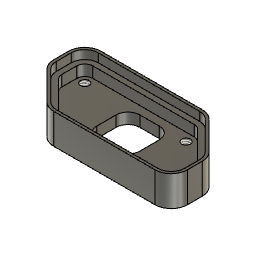
Program and Verify - Challenge (Autodesk Fusion 360 design; units mm, degrees)
Autodesk Fusion 360 part; units mm, degrees
sketch "Sketch1" plane through (0, 0, 0) normal (0, 0, 1) x (1, 0, 0)
  line L0 (47.625, -22.225) -> (-47.625, -22.225)
  line L1 (-47.625, -22.225) -> (-47.625, 22.225)
  line L2 (-47.625, 22.225) -> (47.625, 22.225)
  line L3 (47.625, 22.225) -> (47.625, -22.225)
  line L4 (47.625, -22.225) -> (-47.625, 22.225) construction
  line L5 (-47.625, -22.225) -> (47.625, 22.225) construction
  dimension "d7_1" = 95.25
  dimension "d8_1" = 44.45
  constraint horizontal L0
  constraint perpendicular L0 L1
  constraint parallel L0 L2
  constraint parallel L1 L3
  constraint coincident L4 origin
  constraint coincident L5 origin
  measures "d7_1" distance of L1.end L2.end
  measures "d8_1" distance of L0.end L1.end
extrude "Extrude1" add sketch "Sketch1" along normal blind 17.78
sketch "Sketch2" plane through (0, 0, 17.78) normal (0, 0, 1) x (-1, 0, 0)
  line L0 (-47.625, -22.225) -> (47.625, -22.225)
  line L1 (47.625, -22.225) -> (47.625, 22.225)
  line L2 (47.625, 22.225) -> (-47.625, 22.225)
  line L3 (-47.625, 22.225) -> (-47.625, -22.225)
  line L4 (47.625, 0) -> (25.4, -22.225) construction
  line L5 (-47.625, 0) -> (-25.4, 22.225) construction
  line L6 (47.625, 0) -> (25.4, 22.225)
  line L7 (-47.625, 0) -> (-25.4, -22.225)
  dimension "d11_1" = 45
  dimension "d12_1" = 45
  dimension "d19_1" = 45
  dimension "d20_1" = 45
  constraint midpoint L1 L4.start
  constraint coincident L0 L4.end
  constraint midpoint L3 L5.start
  constraint coincident L2 L5.end
  constraint coincident L2 L6.end
  constraint coincident L0 L7.end
  measures "d11_1" angle of L1 L4
  measures "d12_1" angle of L3 L5
  measures "d19_1" angle of L3 L7
  measures "d20_1" angle of L1 L6
extrude "Extrude2" cut sketch "Sketch2" against normal through all contours L0 L3 L7 | L1 L2 L6
fillet "Fillet1" radius 9.525 6 edges at (-47.625, 0, 8.89) (-25.4, -22.225, 8.89) (47.625, -22.225, 8.89) (47.625, 0, 8.89) (25.4, 22.225, 8.89) (-47.625, 22.225, 8.89)
sketch "Sketch3" plane through (0, 0, 17.78) normal (0, 0, 1) x (-1, 0, 0)
  arc A0 (38.1, -22.225) -> (47.625, -12.7) centre (38.1, -12.7) ccw
  line L0 (47.625, -12.7) -> (47.625, -3.9454)
  arc A1 (47.625, -3.9454) -> (44.8352, 2.7898) centre (38.1, -3.9454) ccw
  line L1 (44.8352, 2.7898) -> (28.1898, 19.4352)
  arc A2 (28.1898, 19.4352) -> (21.4546, 22.225) centre (21.4546, 12.7) ccw
  line L2 (21.4546, 22.225) -> (-38.1, 22.225)
  arc A3 (-38.1, 22.225) -> (-47.625, 12.7) centre (-38.1, 12.7) ccw
  line L3 (-47.625, 12.7) -> (-47.625, 3.9454)
  arc A4 (-47.625, 3.9454) -> (-44.8352, -2.7898) centre (-38.1, 3.9454) ccw
  line L4 (-44.8352, -2.7898) -> (-28.1898, -19.4352)
  arc A5 (-28.1898, -19.4352) -> (-21.4546, -22.225) centre (-21.4546, -12.7) ccw
  line L5 (-21.4546, -22.225) -> (38.1, -22.225)
  line L6 (46.0375, -12.7) -> (46.0375, -3.9454)
  arc A6 (46.0375, -3.9454) -> (43.7127, 1.6673) centre (38.1, -3.9454) ccw
  line L7 (43.7127, 1.6673) -> (27.0673, 18.3127)
  arc A7 (27.0673, 18.3127) -> (21.4546, 20.6375) centre (21.4546, 12.7) ccw
  line L8 (21.4546, 20.6375) -> (-38.1, 20.6375)
  arc A8 (-38.1, 20.6375) -> (-46.0375, 12.7) centre (-38.1, 12.7) ccw
  line L9 (-46.0375, 12.7) -> (-46.0375, 3.9454)
  arc A9 (-46.0375, 3.9454) -> (-43.7127, -1.6673) centre (-38.1, 3.9454) ccw
  line L10 (-43.7127, -1.6673) -> (-27.0673, -18.3127)
  arc A10 (-27.0673, -18.3127) -> (-21.4546, -20.6375) centre (-21.4546, -12.7) ccw
  line L11 (-21.4546, -20.6375) -> (38.1, -20.6375)
  arc A11 (38.1, -20.6375) -> (46.0375, -12.7) centre (38.1, -12.7) ccw
  dimension "d23_1" = -1.5875
extrude "Extrude3" cut sketch "Sketch3" against normal blind 5.08 contours L6 A6 L7 A7 L8 A8 L9 A9 L10 A10 L11 A11
sketch "Sketch4" plane through (0, 0, 12.7) normal (0, 0, 1) x (-1, 0, 0)
  arc A0 (38.1, -20.6375) -> (46.0375, -12.7) centre (38.1, -12.7) ccw
  line L0 (46.0375, -12.7) -> (46.0375, -3.9454)
  arc A1 (46.0375, -3.9454) -> (43.7127, 1.6673) centre (38.1, -3.9454) ccw
  line L1 (43.7127, 1.6673) -> (27.0673, 18.3127)
  arc A2 (27.0673, 18.3127) -> (21.4546, 20.6375) centre (21.4546, 12.7) ccw
  line L2 (21.4546, 20.6375) -> (-38.1, 20.6375)
  arc A3 (-38.1, 20.6375) -> (-46.0375, 12.7) centre (-38.1, 12.7) ccw
  line L3 (-46.0375, 12.7) -> (-46.0375, 3.9454)
  arc A4 (-46.0375, 3.9454) -> (-43.7127, -1.6673) centre (-38.1, 3.9454) ccw
  line L4 (-43.7127, -1.6673) -> (-27.0673, -18.3127)
  arc A5 (-27.0673, -18.3127) -> (-21.4546, -20.6375) centre (-21.4546, -12.7) ccw
  line L5 (-21.4546, -20.6375) -> (38.1, -20.6375)
  line L6 (42.8625, -12.7) -> (42.8625, -3.9454)
  arc A6 (42.8625, -3.9454) -> (41.4676, -0.5778) centre (38.1, -3.9454) ccw
  line L7 (41.4676, -0.5778) -> (24.8222, 16.0676)
  arc A7 (24.8222, 16.0676) -> (21.4546, 17.4625) centre (21.4546, 12.7) ccw
  line L8 (21.4546, 17.4625) -> (-38.1, 17.4625)
  arc A8 (-38.1, 17.4625) -> (-42.8625, 12.7) centre (-38.1, 12.7) ccw
  line L9 (-42.8625, 12.7) -> (-42.8625, 3.9454)
  arc A9 (-42.8625, 3.9454) -> (-41.4676, 0.5778) centre (-38.1, 3.9454) ccw
  line L10 (-41.4676, 0.5778) -> (-24.8222, -16.0676)
  arc A10 (-24.8222, -16.0676) -> (-21.4546, -17.4625) centre (-21.4546, -12.7) ccw
  line L11 (-21.4546, -17.4625) -> (38.1, -17.4625)
  arc A11 (38.1, -17.4625) -> (42.8625, -12.7) centre (38.1, -12.7) ccw
  dimension "d24_1" = -3.175
extrude "Extrude4" cut sketch "Sketch4" against normal blind 6.35 contours L6 A6 L7 A7 L8 A8 L9 A9 L10 A10 L11 A11
sketch "Sketch5" plane through (0, 0, 6.35) normal (0, 0, 1) x (-1, 0, 0)
  arc A0 (38.1, -17.4625) -> (42.8625, -12.7) centre (38.1, -12.7) ccw
  line L0 (42.8625, -12.7) -> (42.8625, -3.9454)
  arc A1 (42.8625, -3.9454) -> (41.4676, -0.5778) centre (38.1, -3.9454) ccw
  line L1 (41.4676, -0.5778) -> (24.8222, 16.0676)
  arc A2 (24.8222, 16.0676) -> (21.4546, 17.4625) centre (21.4546, 12.7) ccw
  line L2 (21.4546, 17.4625) -> (-38.1, 17.4625)
  arc A3 (-38.1, 17.4625) -> (-42.8625, 12.7) centre (-38.1, 12.7) ccw
  line L3 (-42.8625, 12.7) -> (-42.8625, 3.9454)
  arc A4 (-42.8625, 3.9454) -> (-41.4676, 0.5778) centre (-38.1, 3.9454) ccw
  line L4 (-41.4676, 0.5778) -> (-24.8222, -16.0676)
  arc A5 (-24.8222, -16.0676) -> (-21.4546, -17.4625) centre (-21.4546, -12.7) ccw
  line L5 (-21.4546, -17.4625) -> (38.1, -17.4625)
  point P0 (38.1, -12.7)
  point P1 (25.4, -12.7)
  point P2 (12.7, -12.7)
  point P3 (0, -12.7)
  point P4 (-12.7, -12.7)
  point P5 (25.4, 0)
  point P6 (12.7, 0)
  point P7 (-12.7, 0)
  point P8 (-25.4, 0)
  point P9 (12.7, 12.7)
  point P10 (0, 12.7)
  point P11 (-12.7, 12.7)
  point P12 (-25.4, 12.7)
  point P13 (-38.1, 12.7)
  point P14 (-21.4546, -12.7)
  point P15 (21.4546, 12.7)
  dimension "d27_1" = 12.7
  dimension "d28_1" = 12.7
  dimension "d29_1" = 12.7
  dimension "d30_1" = 12.7
  constraint coincident P0 A0.centre
  constraint coincident P13 A3.centre
  constraint horizontal P12 P13
  constraint horizontal P11 P12
  constraint horizontal P10 P11
  constraint horizontal P9 P10
  constraint vertical P8 P12
  constraint vertical P7 P11
  constraint vertical origin P10
  constraint vertical P6 P9
  constraint horizontal P5 P6
  constraint horizontal origin P6
  constraint horizontal origin P7
  constraint horizontal P7 P8
  constraint horizontal P0 P1
  constraint horizontal P1 P2
  constraint horizontal P2 P3
  constraint horizontal P3 P4
  constraint vertical P1 P5
  constraint vertical P2 P6
  constraint vertical P3 origin
  constraint vertical P4 P7
  constraint coincident P14 A5.centre
  constraint coincident P15 A2.centre
  measures "d27_1" distance of P12 P13
  measures "d28_1" distance of P11 P12
  measures "d29_1" distance of P9 P10
  measures "d30_1" distance of P5 P6
hole "Hole2" at (-38.1, 12.7, 6.35) at (21.4546, 12.7, 6.35) at (38.1, -12.7, 6.35) at (-21.4546, -12.7, 6.35) direction (0, 0, -1) diameter 5.1308 end through all
thread "Thread2" "ANSI Unified Screw Threads 0.25 1/4-20 UNC 1B"
sketch "Sketch7" plane through (0, 0, 6.35) normal (0, 0, 1) x (-1, 0, 0)
  circle A0 centre (-38.1, 12.7) radius 2.5591
  circle A1 centre (38.1, -12.7) radius 2.5591
  circle A2 centre (-21.4546, -12.7) radius 2.5591
  circle A3 centre (21.4546, 12.7) radius 2.5591
  arc A4 (38.1, -17.4625) -> (42.8625, -12.7) centre (38.1, -12.7) ccw
  line L0 (42.8625, -12.7) -> (42.8625, -3.9454)
  arc A5 (42.8625, -3.9454) -> (41.4676, -0.5778) centre (38.1, -3.9454) ccw
  line L1 (41.4676, -0.5778) -> (24.8222, 16.0676)
  arc A6 (24.8222, 16.0676) -> (21.4546, 17.4625) centre (21.4546, 12.7) ccw
  line L2 (21.4546, 17.4625) -> (-38.1, 17.4625)
  arc A7 (-38.1, 17.4625) -> (-42.8625, 12.7) centre (-38.1, 12.7) ccw
  line L3 (-42.8625, 12.7) -> (-42.8625, 3.9454)
  arc A8 (-42.8625, 3.9454) -> (-41.4676, 0.5778) centre (-38.1, 3.9454) ccw
  line L4 (-41.4676, 0.5778) -> (-24.8222, -16.0676)
  arc A9 (-24.8222, -16.0676) -> (-21.4546, -17.4625) centre (-21.4546, -12.7) ccw
  line L5 (-21.4546, -17.4625) -> (38.1, -17.4625)
  line L6 (-12.7, 12.7) -> (12.7, 12.7)
  line L7 (12.7, 12.7) -> (12.7, -12.7)
  line L8 (12.7, -12.7) -> (-12.7, -12.7)
  line L9 (-12.7, -12.7) -> (-12.7, 12.7)
  line L10 (-12.7, 12.7) -> (12.7, -12.7) construction
  line L11 (12.7, 12.7) -> (-12.7, -12.7) construction
  dimension "d54_1" = 25.4
  dimension "d55_1" = 25.4
  constraint horizontal L6
  constraint perpendicular L6 L7
  constraint parallel L6 L8
  constraint parallel L7 L9
  constraint coincident L10 origin
  constraint coincident L11 origin
  measures "d54_1" distance of L7.end L8.end
  measures "d55_1" distance of L6.end L7.end
extrude "Extrude6" cut sketch "Sketch7" against normal through all contours L6 L7 L8 L9
fillet "Fillet3" radius 6.985 4 edges at (-12.7, 12.7, 3.175) (12.7, 12.7, 3.175) (12.7, -12.7, 3.175) (-12.7, -12.7, 3.175)
equation "d28_1 = d27_1"
equation "d29_1 = d27_1"
equation "d30_1 = d27_1"
